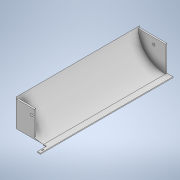
# Autodesk Inventor part: 22
Saved by Autodesk Inventor 2020 (Build 240168000, 168)
## iProperties
Created: 2020-12-03
Part Number: 22
Material: 常规
Document SubType Name: Sheet Metal
Designer: huang
Density: 1 g/cm^3
Sheet Metal Rule: 默认_mm
Appearance: 默认
Author: huang
Autodesk Inventor part; units mm, degrees
ref_plane "YZ Plane" through (0, 0, 0) normal (1, 0, 0) x (0, 1, 0)
ref_plane "XZ Plane" through (0, 0, 0) normal (0, 1, 0) x (-1, 0, 0)
ref_plane "XY Plane" through (0, 0, 0) normal (0, 0, 1) x (1, 0, 0)
sketch "草图1" plane through (0, 0, 0) normal (0, 1, 0) x (-1, 0, 0)
  line L0 (44.8045, 690.8377) -> (-45.1955, 690.8377)
  line L1 (-45.1955, 690.8377) -> (-45.1955, -101.1623)
  line L2 (-45.1955, -101.1623) -> (44.8045, -101.1623)
  line L3 (44.8045, -101.1623) -> (44.8045, 690.8377)
  point P0 (0, 0)
  dimension "d0" = 90
  dimension "d1" = 792
  constraints: 8 end point, 2 parallel, 1 horizontal, 1 perpendicular
  measures "d0" distance of L1.end L2.end
  measures "d1" distance of L2.end L0.start
extrude "拉伸1" add sketch "草图1" along normal blind 90
sketch "草图3" plane through (-44.8045, 0, 690.8377) normal (0, 0, 1) x (1, 0, 0)
  line L0 (90, 0) -> (90, 90) projected
  circle A0 centre (90, 90) radius 90
  line L1 (0, 0) -> (0, 90) projected
  point P0 (44.8045, 0)
  constraints: 1 horizontal alignment, 1 vertical, 1 other
extrude "拉伸3" cut sketch "草图3" against normal through all
sketch "草图6" plane through (-44.8045, 0, 690.8377) normal (0, 0, 1) x (1, 0, 0)
  line L0 (0, 0) -> (0, 90) projected
  line L1 (0, 0) -> (90, 0) projected
  arc A0 (0, 90) -> (90, 0) centre (90, 90) ccw
  arc A1 (0, 90) -> (90, 0) centre (90, 90) ccw projected
  line L2 (0, 90) -> (0, 0)
  line L3 (0, 0) -> (90, 0)
  constraints: 4 end point, 2 point on circle, 1 centre point, 1 concentric, 1 vertical
extrude "拉伸6" cut sketch "草图6" against normal blind 386
sketch "草图9" plane through (0, 0, 0) normal (0, -1, 0) x (1, 0, 0)
  line L0 (45.1955, -101.1623) -> (-44.8045, -101.1623) projected
  line L1 (45.1955, 304.8377) -> (45.1955, -101.1623) projected
  line L2 (-44.8045, -101.1623) -> (45.1955, -101.1623)
  line L3 (45.1955, -101.1623) -> (45.1955, -96.1623)
  line L4 (45.1955, -96.1623) -> (-44.8045, -96.1623)
  line L5 (-44.8045, -96.1623) -> (-44.8045, -101.1623)
  point P0 (0, 0)
  point P1 (43.3955, 107.8377)
  point P2 (-44.8045, 304.8377)
  dimension "d75" = 5
  constraints: 8 end point, 2 parallel, 1 horizontal, 1 perpendicular, 1 point on line
  measures "d75" distance between parallel lines of L0 L4
extrude "拉伸9" add sketch "草图9" against normal blind 85
sketch "草图12" plane through (0, 0, 0) normal (0, -1, 0) x (1, 0, 0)
  line L0 (-44.8045, -101.1623) -> (-44.8045, 304.8377) projected
  line L1 (-44.8045, 304.8377) -> (15.1955, 304.8377)
  line L2 (15.1955, 304.8377) -> (15.1955, 299.8377)
  line L3 (15.1955, 299.8377) -> (-44.8045, 299.8377)
  line L4 (-44.8045, 299.8377) -> (-44.8045, 304.8377)
  point P0 (0, 0)
  point P1 (45.1955, 304.8377)
  dimension "d76" = 5
  dimension "d77" = 60
  constraints: 8 end point, 2 parallel, 1 horizontal, 1 perpendicular
  measures "d76" distance of L1.end L2.end
  measures "d77" distance of L2.end L3.end
extrude "拉伸12" add sketch "草图12" against normal blind 85
sketch "草图13" plane through (-44.8045, 0, 304.8377) normal (0, 0, 1) x (1, 0, 0)
  line L0 (60, 5.1472) -> (60, 85) projected
  line L1 (60, 85) -> (60, 65)
  line L2 (60, 65) -> (52, 65)
  circle A0 centre (52, 65) radius 4
  point P0 (44.8045, 0)
  point P1 (50, 85)
  dimension "d81" = 20
  dimension "d82" = 8
  dimension "d83" = 8
  constraints: 4 end point, 1 centre point, 1 coincident, 1 perpendicular, 1 point on line
  measures "d81" distance of L0.end L1.end
  measures "d82" distance of L1.end L2.end
  measures "d83" diameter of A0
extrude "拉伸13" cut sketch "草图13" against normal blind 1000
sketch "草图20" plane through (45.1955, 0, -96.1623) normal (1, 0, 0) x (0, 0, -1)
  line L0 (5, 0) -> (5, 85) projected
  line L1 (5, 0) -> (-401, 0)
  line L2 (-401, 0) -> (-401, -3)
  line L3 (-401, -3) -> (5, -3)
  line L4 (5, -3) -> (5, 0)
  point P0 (-96.1623, 0)
  dimension "d84" = 3
  constraints: 8 end point, 2 parallel, 1 horizontal, 1 perpendicular
  measures "d84" distance of L1.end L2.end
extrude "拉伸20" add sketch "草图20" along normal blind 20
sketch "草图21" plane through (45.1955, -3, 304.8377) normal (0, 0, 1) x (1, 0, 0)
  line L0 (20, 3) -> (10, 3)
  line L1 (10, 3) -> (10, 0)
  line L2 (10, 0) -> (20, 0)
  line L3 (20, 0) -> (20, 3)
  point P0 (-45.1955, 3)
  dimension "d87" = 10
  dimension "d97" = 3
  constraints: 8 end point, 2 parallel, 1 horizontal, 1 perpendicular
  measures "d87" distance of L1.end L2.end
  measures "d97" distance of L0.end L1.end
extrude "拉伸21" add sketch "草图21" along normal blind 30
sketch "草图22" plane through (45.1955, 0, -101.1623) normal (0, 1, 0) x (1, 0, 0)
  circle A0 centre (14.5, -425.4) radius 1.5
  line L0 (20, -436) -> (10, -436) projected
  line L1 (20, 0) -> (20, -436) projected
  line L2 (14.5, -425.4) -> (14.5, -421.4)
  circle A1 centre (14.5, -421.4) radius 1.5
  point P0 (-45.1955, -101.1623)
  dimension "d90" = 3
  dimension "d93" = 10.6
  dimension "d94" = 5.5
  dimension "d95" = 4
  dimension "d96" = 3
  constraints: 2 centre point, 2 end point, 1 coincident
  measures "d90" diameter of A0
  measures "d93" distance from line of L0 L2.start
  measures "d94" distance from line of L1 L2.start
  measures "d95" distance of L2.start L2.end
  measures "d96" diameter of A1
extrude "拉伸22" cut sketch "草图22" against normal blind 30
equation "\"折弯半径\" = 厚度"
equation "\"折弯释压宽度\" = 厚度"
equation "\"折弯释压深度\" = 0.5 * 厚度"
equation "\"拐角释压尺寸\" = 4 * 厚度"
equation "\"最小余量\" = 2 * 厚度"
equation "\"过渡半径\" = 折弯半径"
equation "\"Jacobi半径尺寸\" = 折弯半径"
equation "\"间隙大小\" = 厚度"
equation "\"厚度\" = 0.5"
